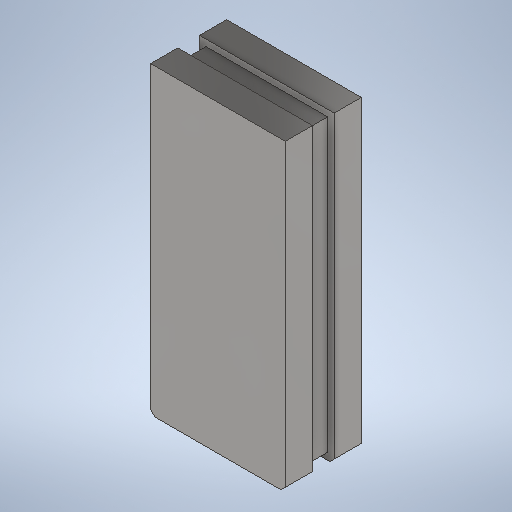
# Autodesk Inventor part: lmGUIDE
Saved by Autodesk Inventor 2025 (Build 290162000, 162)
## iProperties
Created: 2024-12-23
Part Number: lmGUIDE
Material: Generic
Document SubType Name: Modeling
Designer: DMIADX
Density: 1 g/cm^3
Appearance: Steel - Polished
Author: DMIADX
Autodesk Inventor part; units mm, degrees
ref_plane "YZ Plane" through (0, 0, 0) normal (1, 0, 0) x (0, 1, 0)
ref_plane "XZ Plane" through (0, 0, 0) normal (0, 1, 0) x (-1, 0, 0)
ref_plane "XY Plane" through (0, 0, 0) normal (0, 0, 1) x (1, 0, 0)
sketch "Sketch1" plane through (0, 0, 0) normal (0, 0, 1) x (1, 0, 0)
  line L0 (29, -70) -> (-29, -70)
  line L1 (-31, -68) -> (-31, 70)
  line L2 (-31, 70) -> (31, 70)
  line L3 (31, 70) -> (31, -68)
  line L4 (31, -70) -> (-31, 70) construction
  line L5 (-31, -70) -> (31, 70) construction
  line L6 (-31, -68) -> (-29, -70)
  line L7 (29, -70) -> (31, -68)
  line L8 (-28, 67) -> (-28, -66.7574)
  line L9 (-28, -66.7574) -> (-27.7574, -67)
  line L10 (-27.7574, -67) -> (27.7574, -67)
  line L11 (27.7574, -67) -> (28, -66.7574)
  line L12 (28, -66.7574) -> (28, 67)
  line L13 (28, 67) -> (-28, 67)
  point P0 (0, 0)
  dimension "d0" = 62
  dimension "d1" = 140
  dimension "d2" = 2
  dimension "d3" = 2
  dimension "d4" = 2
  dimension "d5" = 2
  dimension "d6" = 3
  constraints: 28 end point, 4 parallel, 4 point on line, 2 midpoint, 2 perpendicular, 1 horizontal, 5 other
  measures "d0" distance of L1.end L2.end
  measures "d1" distance of L5.start L1.end
  measures "d2" distance of L1.start L5.start
  measures "d3" distance of L0.end L5.start
  measures "d4" distance of L0.start L4.start
  measures "d5" distance of L3.end L4.start
  measures "d6" distance between parallel lines of L1 L8
extrude "Extrusion1" add sketch "Sketch1" along normal mid plane 35 contours L0 L6 L1 L2 L3 L7 | L13 L12 L11 L10 L9 L8
extrude "Extrusion2" cut sketch "Sketch1" along normal mid plane 10
sketch "Sketch2" plane through (-31, -68, -17.5) normal (-1, 0, 0) x (0, 0, 1)
  line L0 (2, 30) -> (2, 44.8794) construction
  line L1 (2, 44.8794) -> (5.048, 44.8794) construction
  line L2 (5.048, 44.8794) -> (5.048, 30) construction
  line L3 (5.048, 30) -> (2, 30) construction
  line L4 (0, 0) -> (0, 138) projected
  spline S0 degree 2 poles (5.0549, 35.4277) (5.8904, 35.4277) (7.2349, 34.7505) (7.6106, 34.182) knots 0 0 0 1 2 2 2
  spline S1 degree 2 poles (7.6106, 34.182) (7.9023, 33.7173) (8.1, 32.7633) (8.1, 32.0218) knots 0 0 0 1 2 2 2
  line L5 (8.1, 32.0218) -> (8.1, 30.6179)
  line L6 (8.1, 30.6179) -> (2, 30.6179)
  line L7 (2, 30.6179) -> (2, 32.007)
  spline S2 degree 2 poles (2, 32.007) (2, 32.8671) (2.2571, 33.8459) (2.4844, 34.1919) knots 0 0 0 1 2 2 2
  spline S3 degree 2 poles (2.4844, 34.1919) (2.875, 34.7801) (4.1652, 35.4277) (5.0549, 35.4277) knots 0 0 0 1 2 2 2
  spline S4 degree 2 poles (5.0451, 34.5824) (4.3431, 34.5824) (3.3495, 34.1177) (3.0677, 33.658) knots 0 0 0 1 2 2 2
  spline S5 degree 2 poles (3.0677, 33.658) (2.875, 33.3318) (2.7019, 32.5952) (2.7019, 32.0465) knots 0 0 0 1 2 2 2
  line L8 (2.7019, 32.0465) -> (2.7019, 31.4286)
  line L9 (2.7019, 31.4286) -> (7.3981, 31.4286)
  line L10 (7.3981, 31.4286) -> (7.3981, 32.0465)
  spline S6 degree 2 poles (7.3981, 32.0465) (7.3981, 32.5853) (7.225, 33.401) (6.9927, 33.7322) knots 0 0 0 1 2 2 2
  spline S7 degree 2 poles (6.9927, 33.7322) (6.706, 34.1573) (5.7569, 34.5824) (5.0451, 34.5824) knots 0 0 0 1 2 2 2
  line L11 (8.1, 41.5376) -> (8.1, 40.7269)
  line L12 (8.1, 40.7269) -> (2.8453, 40.7269)
  line L13 (2.8453, 40.7269) -> (6.4193, 39.1352)
  line L14 (6.4193, 39.1352) -> (6.4193, 38.6408)
  line L15 (6.4193, 38.6408) -> (2.8453, 37.0639)
  line L16 (2.8453, 37.0639) -> (8.1, 37.0639)
  line L17 (8.1, 37.0639) -> (8.1, 36.3076)
  line L18 (8.1, 36.3076) -> (2, 36.3076)
  line L19 (2, 36.3076) -> (2, 37.4149)
  line L20 (2, 37.4149) -> (5.396, 38.9374)
  line L21 (5.396, 38.9374) -> (2, 40.4105)
  line L22 (2, 40.4105) -> (2, 41.5376)
  line L23 (2, 41.5376) -> (8.1, 41.5376)
  line L24 (8.1, 44.899) -> (8.1, 42.5361)
  line L25 (8.1, 42.5361) -> (7.4771, 42.5361)
  line L26 (7.4771, 42.5361) -> (7.4771, 43.3122)
  line L27 (7.4771, 43.3122) -> (2.6229, 43.3122)
  line L28 (2.6229, 43.3122) -> (2.6229, 42.5361)
  line L29 (2.6229, 42.5361) -> (2, 42.5361)
  line L30 (2, 42.5361) -> (2, 44.899)
  line L31 (2, 44.899) -> (2.6229, 44.899)
  line L32 (2.6229, 44.899) -> (2.6229, 44.1229)
  line L33 (2.6229, 44.1229) -> (7.4771, 44.1229)
  line L34 (7.4771, 44.1229) -> (7.4771, 44.899)
  line L35 (7.4771, 44.899) -> (8.1, 44.899)
  line L36 (8.1, 45.2451) -> (2, 47.3015)
  line L37 (2, 47.3015) -> (2, 48.3)
  line L38 (2, 48.3) -> (8.1, 50.3564)
  line L39 (8.1, 50.3564) -> (8.1, 49.5012)
  line L40 (8.1, 49.5012) -> (6.3946, 48.9476)
  line L41 (6.3946, 48.9476) -> (6.3946, 46.6193)
  line L42 (6.3946, 46.6193) -> (8.1, 46.0656)
  line L43 (8.1, 46.0656) -> (8.1, 45.2451)
  line L44 (5.7025, 48.7251) -> (2.8305, 47.781)
  line L45 (2.8305, 47.781) -> (5.7025, 46.8417)
  line L46 (5.7025, 46.8417) -> (5.7025, 48.7251)
  point P0 (17.5, 68)
  dimension "d11" = 2
  dimension "d12" = 30
  constraints: 2 other
  measures "d11" distance from line of L4 L0.start
  measures "d12" vertical distance of L4.start L0.start
emboss "Emboss1" sketch "Sketch2" operation cut depth 1 direction (1, 0, 0)
equation "\"d3\" = d2"
equation "\"d4\" = d2"
equation "\"d5\" = d4"
body "Solid1"
